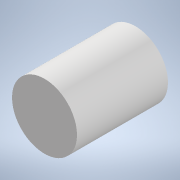
# Autodesk Inventor part: PotAttachmentB10R
Saved by Autodesk Inventor 2022 (Build 260153000, 153)
## iProperties
Created: 2021-12-04
Part Number: PotAttachmentB10R
Material: Generic
Document SubType Name: Modeling
Designer: teh18
Density: 1 g/cm^3
Appearance: Default
Author: teh18
Autodesk Inventor part; units mm, degrees
ref_plane "YZ Plane" through (0, 0, 0) normal (1, 0, 0) x (0, 1, 0)
ref_plane "XZ Plane" through (0, 0, 0) normal (0, 1, 0) x (-1, 0, 0)
ref_plane "Work Plane1" through (-2.5858, -0.1842, 12) normal (0, 0, 1) x (1, 0, 0)
sketch "Sketch1" plane through (0, 0, 0) normal (0, 0, 1) x (1, 0, 0)
  line L0 (-1.7235, 1.3627) -> (-1.9283, 2.2145) projected
  arc A0 (-1.9283, 2.2145) -> (-2.598, 1.4164) centre (0.0001, -0.0836) ccw projected
  line L1 (-2.598, 1.4164) -> (-1.7235, 1.3627) projected
  line L2 (-1.1249, 1.865) -> (-1.026, 2.7355) projected
  arc A1 (-1.026, 2.7355) -> (-1.9283, 2.2145) centre (0.0001, -0.0836) ccw projected
  line L3 (-1.9283, 2.2145) -> (-1.1249, 1.865) projected
  line L4 (-0.3906, 2.1322) -> (0.0001, 2.9164) projected
  arc A2 (0.0001, 2.9164) -> (-1.026, 2.7355) centre (0.0001, -0.0836) ccw projected
  line L5 (-1.026, 2.7355) -> (-0.3906, 2.1322) projected
  line L6 (0.3908, 2.1322) -> (1.0261, 2.7355) projected
  arc A3 (1.0261, 2.7355) -> (0.0001, 2.9164) centre (0.0001, -0.0836) ccw projected
  line L7 (0.0001, 2.9164) -> (0.3908, 2.1322) projected
  line L8 (1.0261, 2.7355) -> (1.1251, 1.865) projected
  line L9 (1.1251, 1.865) -> (1.9284, 2.2145) projected
  arc A4 (1.9284, 2.2145) -> (1.0261, 2.7355) centre (0.0001, -0.0836) ccw projected
  line L10 (1.9284, 2.2145) -> (1.7237, 1.3627) projected
  line L11 (1.7237, 1.3627) -> (2.5982, 1.4164) projected
  arc A5 (2.5982, 1.4164) -> (1.9284, 2.2145) centre (0.0001, -0.0836) ccw projected
  line L12 (2.5982, 1.4164) -> (2.1144, 0.6859) projected
  line L13 (2.1144, 0.6859) -> (2.9545, 0.4373) projected
  arc A6 (2.9545, 0.4373) -> (2.5982, 1.4164) centre (0.0001, -0.0836) ccw projected
  line L14 (-2.9543, -0.6046) -> (-2.926, -0.5836) projected
  line L15 (-2.926, -0.5836) -> (2.9262, -0.5836) projected
  line L16 (2.9262, -0.5836) -> (2.9545, -0.6046) projected
  arc A7 (2.9545, -0.6046) -> (2.9545, 0.4373) centre (0.0001, -0.0836) ccw projected
  line L17 (2.9545, 0.4373) -> (2.9262, 0.4164) projected
  line L18 (2.9262, 0.4164) -> (-2.926, 0.4164) projected
  line L19 (-2.926, 0.4164) -> (-2.9543, 0.4373) projected
  arc A8 (-2.9543, 0.4373) -> (-2.9543, -0.6046) centre (0.0001, -0.0836) ccw projected
  line L20 (2.9545, -0.6046) -> (2.1144, -0.8532) projected
  line L21 (2.1144, -0.8532) -> (2.5982, -1.5836) projected
  arc A9 (2.5982, -1.5836) -> (2.9545, -0.6046) centre (0.0001, -0.0836) ccw projected
  line L22 (2.5982, -1.5836) -> (1.7237, -1.5299) projected
  line L23 (1.7237, -1.5299) -> (1.9284, -2.3817) projected
  arc A10 (1.9284, -2.3817) -> (2.5982, -1.5836) centre (0.0001, -0.0836) ccw projected
  line L24 (1.1251, -2.0322) -> (1.0261, -2.9027) projected
  arc A11 (1.0261, -2.9027) -> (1.9284, -2.3817) centre (0.0001, -0.0836) ccw projected
  line L25 (1.9284, -2.3817) -> (1.1251, -2.0322) projected
  line L26 (0.3908, -2.2994) -> (0.0001, -3.0836) projected
  arc A12 (0.0001, -3.0836) -> (1.0261, -2.9027) centre (0.0001, -0.0836) ccw projected
  line L27 (1.0261, -2.9027) -> (0.3908, -2.2994) projected
  line L28 (-0.3906, -2.2994) -> (-1.026, -2.9027) projected
  arc A13 (-1.026, -2.9027) -> (0.0001, -3.0836) centre (0.0001, -0.0836) ccw projected
  line L29 (0.0001, -3.0836) -> (-0.3906, -2.2994) projected
  line L30 (-1.1249, -2.0322) -> (-1.9283, -2.3817) projected
  arc A14 (-1.9283, -2.3817) -> (-1.026, -2.9027) centre (0.0001, -0.0836) ccw projected
  line L31 (-1.026, -2.9027) -> (-1.1249, -2.0322) projected
  line L32 (-1.7235, -1.5299) -> (-2.598, -1.5836) projected
  arc A15 (-2.598, -1.5836) -> (-1.9283, -2.3817) centre (0.0001, -0.0836) ccw projected
  line L33 (-1.9283, -2.3817) -> (-1.7235, -1.5299) projected
  line L34 (-2.598, -1.5836) -> (-2.1142, -0.8532) projected
  line L35 (-2.1142, -0.8532) -> (-2.9543, -0.6046) projected
  arc A16 (-2.9543, -0.6046) -> (-2.598, -1.5836) centre (0.0001, -0.0836) ccw projected
  line L36 (-2.9543, 0.4373) -> (-2.1142, 0.6859) projected
  line L37 (-2.1142, 0.6859) -> (-2.598, 1.4164) projected
  arc A17 (-2.598, 1.4164) -> (-2.9543, 0.4373) centre (0.0001, -0.0836) ccw projected
  circle A18 centre (0.0001, -0.0836) radius 5
  point P0 (0, 0)
  dimension "d2" = 10
  constraints: 1 centre point, 1 coincident
  measures "d2" diameter of A18
extrude "Extrusion1" add sketch "Sketch1" along normal up to surface (12 mm away) contours L19 L18 L17 A7 L16 L15 L14 A8 | A18
sketch "Sketch2" plane through (0.0001, -0.0836, 12) normal (0, 0, 1) x (1, 0, 0)
  line L0 (-92.2971, 80.1427) -> (-95.7176, 83.0515) projected
  line L1 (-95.7176, 83.0515) -> (-97.1769, 81.3355) projected
  line L2 (-97.1769, 81.3355) -> (-94.5854, 79.1317) projected
  spline S0 degree 2 poles (-94.5854, 79.1317) (-94.0347, 78.6633) (-94.508, 78.1067) knots 0 0 0 1 1 1 projected
  spline S1 degree 2 poles (-94.508, 78.1067) (-94.9862, 77.5444) (-95.537, 78.0128) knots 0 0 0 1 1 1 projected
  line L3 (-95.537, 78.0128) -> (-98.1284, 80.2166) projected
  line L4 (-98.1284, 80.2166) -> (-100.7119, 77.1787) projected
  spline S2 degree 2 poles (-100.7119, 77.1787) (-101.1999, 76.6047) (-101.7391, 77.0633) knots 0 0 0 1 1 1 projected
  spline S3 degree 2 poles (-101.7391, 77.0633) (-102.2899, 77.5316) (-101.8018, 78.1056) knots 0 0 0 1 1 1 projected
  line L5 (-101.8018, 78.1056) -> (-95.8559, 85.0973) projected
  line L6 (-95.8559, 85.0973) -> (-91.3455, 81.2616) projected
  spline S4 degree 2 poles (-91.3455, 81.2616) (-90.7948, 80.7932) (-91.2681, 80.2367) knots 0 0 0 1 1 1 projected
  spline S5 degree 2 poles (-91.2681, 80.2367) (-91.7463, 79.6743) (-92.2971, 80.1427) knots 0 0 0 1 1 1 projected
  spline S6 degree 2 poles (-106.1381, 87.2679) (-104.8415, 88.7926) (-103.1653, 89.2952) knots 0 0 0 1 1 1 projected
  spline S7 degree 2 poles (-103.1653, 89.2952) (-101.3052, 89.8613) (-100.053, 88.7964) knots 0 0 0 1 1 1 projected
  spline S8 degree 2 poles (-100.053, 88.7964) (-98.7138, 87.6575) (-98.905, 85.6822) knots 0 0 0 1 1 1 projected
  spline S9 degree 2 poles (-98.905, 85.6822) (-99.0904, 83.9018) (-100.3871, 82.3771) knots 0 0 0 1 1 1 projected
  spline S10 degree 2 poles (-100.3871, 82.3771) (-101.6886, 80.8466) (-103.2555, 80.4607) knots 0 0 0 1 1 1 projected
  spline S11 degree 2 poles (-103.2555, 80.4607) (-105.2005, 79.877) (-106.4933, 80.9764) knots 0 0 0 1 1 1 projected
  spline S12 degree 2 poles (-106.4933, 80.9764) (-107.792, 82.0808) (-107.6005, 83.9859) knots 0 0 0 1 1 1 projected
  spline S13 degree 2 poles (-107.6005, 83.9859) (-107.4348, 85.7431) (-106.1381, 87.2679) knots 0 0 0 1 1 1 projected
  line L7 (-91.7338, 74.7785) -> (-94.3173, 71.7407) projected
  spline S14 degree 2 poles (-94.3173, 71.7407) (-94.8053, 71.1667) (-95.3445, 71.6252) knots 0 0 0 1 1 1 projected
  spline S15 degree 2 poles (-95.3445, 71.6252) (-95.8953, 72.0936) (-95.4072, 72.6676) knots 0 0 0 1 1 1 projected
  line L8 (-95.4072, 72.6676) -> (-89.4614, 79.6593) projected
  line L9 (-89.4614, 79.6593) -> (-84.9509, 75.8236) projected
  spline S16 degree 2 poles (-84.9509, 75.8236) (-84.4002, 75.3552) (-84.8735, 74.7987) knots 0 0 0 1 1 1 projected
  spline S17 degree 2 poles (-84.8735, 74.7987) (-85.3517, 74.2363) (-85.9025, 74.7047) knots 0 0 0 1 1 1 projected
  line L10 (-85.9025, 74.7047) -> (-89.323, 77.6135) projected
  line L11 (-89.323, 77.6135) -> (-90.7823, 75.8975) projected
  line L12 (-90.7823, 75.8975) -> (-88.1908, 73.6937) projected
  spline S18 degree 2 poles (-88.1908, 73.6937) (-87.6401, 73.2253) (-88.1134, 72.6687) knots 0 0 0 1 1 1 projected
  spline S19 degree 2 poles (-88.1134, 72.6687) (-88.5916, 72.1064) (-89.1424, 72.5747) knots 0 0 0 1 1 1 projected
  line L13 (-89.1424, 72.5747) -> (-91.7338, 74.7785) projected
  line L14 (13.2434, -3.5653) -> (42.3957, 30.7151) projected
  line L15 (42.3957, 30.7151) -> (-82.2993, 136.7567) projected
  line L16 (-82.2993, 136.7567) -> (-130.8864, 79.6227) projected
  ellipse E0 centre (-123.2395, 73.1197) end of major axis (-130.8864, 79.6227) minor radius 10 (-130.8864, 79.6227) -> (-129.7178, 65.5018) ccw projected
  line L17 (-129.7178, 65.5018) -> (-126.9376, 63.1376) projected
  arc A0 (-146.3725, 40.284) -> (-126.9376, 63.1376) centre (-127.0356, 43.5304) ccw projected
  line L18 (-146.3725, 40.284) -> (-149.1526, 42.6483) projected
  ellipse E1 centre (-155.6309, 35.0304) end of major axis (-163.2779, 41.5334) minor radius 10 (-149.1526, 42.6483) -> (-163.2779, 41.5334) ccw projected
  line L19 (-163.2779, 41.5334) -> (-185.9519, 14.8709) projected
  line L20 (-185.9519, 14.8709) -> (-114.5819, -45.8226) projected
  line L21 (-114.5819, -45.8226) -> (-63.4034, 14.3584) projected
  arc A1 (-19.6407, 24.3997) -> (-63.4034, 14.3584) centre (-45.2642, 35.6885) ccw projected
  line L22 (-19.6407, 24.3997) -> (13.2434, -3.5653) projected
  circle A2 centre (-78.021, 63.5451) radius 2.4 projected
  circle A3 centre (-59.7041, 76.1914) radius 2.4 projected
  circle A4 centre (-37.5181, 77.985) radius 2.4 projected
  circle A5 centre (-17.4076, 68.4452) radius 2.4 projected
  circle A6 centre (0, 0) radius 5 projected
  point P0 (-0.0001, 0.0836)
  constraints: 2 other
extrude "Extrusion2" add sketch "Sketch2" along normal blind 2 contours A6
thicken "Thicken2" operation add thickness 0.2 both sides no extend neighbours yes toward (-0.8459864, -0.5332044, 0) faces at (-2.5379, -1.6832, 8)
thicken "Thicken3" operation add thickness 0.2 both sides no extend neighbours yes toward (0.96839, 0.2494411, 0) faces at (2.9052, 0.6647, 8)
spur gear teeth "Spur Gear1" teeth 30 pitch diameter 30 tip diameter 32 root diameter 27.5 face width 14 trims to tip circle yes start plane through (0.0001, -0.0836, 0) normal (0, 0, -1) x (-1, 0, 0)
body "Solid1"
